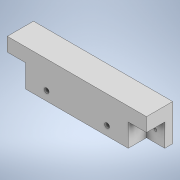
# Autodesk Inventor part: side_bumper_upper
Saved by Autodesk Inventor 2020 (Build 240168000, 168)
## iProperties
Created: 2022-07-20
Part Number: side_bumper_upper
Material: 일반
Document SubType Name: Modeling
Designer: SeungJin
Density: 1 g/cm^3
Appearance: 기본값
Author: SeungJin
Autodesk Inventor part; units mm, degrees
ref_plane "YZ Plane" through (0, 0, 0) normal (1, 0, 0) x (0, 1, 0)
ref_plane "XZ Plane" through (0, 0, 0) normal (0, 1, 0) x (-1, 0, 0)
ref_plane "XY Plane" through (0, 0, 0) normal (0, 0, 1) x (1, 0, 0)
ref_plane "작업 평면1" through (-180.5399, 22.5444, -43) normal (0, 0, 1) x (1, 0, 0)
sketch "스케치3" plane through (-180.5399, 22.5444, -43) normal (0, 0, 1) x (1, 0, 0)
  line L0 (146.4615, -22.6) -> (144.383, -19) projected
  line L1 (144.383, -19) -> (146.4615, -15.4) projected
  line L2 (146.4615, -15.4) -> (150.6184, -15.4) projected
  line L3 (150.6184, -15.4) -> (152.6968, -19) projected
  line L4 (152.6968, -19) -> (150.6184, -22.6) projected
  line L5 (150.6184, -22.6) -> (146.4615, -22.6) projected
  line L6 (45.113, -19) -> (47.1915, -15.4) projected
  line L7 (47.1915, -15.4) -> (51.3484, -15.4) projected
  line L8 (51.3484, -15.4) -> (53.4269, -19) projected
  line L9 (53.4269, -19) -> (51.3484, -22.6) projected
  line L10 (51.3484, -22.6) -> (47.1915, -22.6) projected
  line L11 (47.1915, -22.6) -> (45.113, -19) projected
  circle A0 centre (34.635, -45) radius 2.25 projected
  circle A1 centre (133.9049, -45) radius 2.25 projected
  line L12 (168.5399, -60) -> (0, -60) projected
  line L13 (198.5399, -22.5444) -> (168.5399, -22.5444) projected
  line L14 (168.5399, -22.5444) -> (168.5399, -60) projected
  line L15 (198.5399, 0) -> (198.5399, -22.5444) projected
  line L16 (0, 0) -> (198.5399, 0) projected
  line L17 (0, -60) -> (0, 0) projected
  line L18 (0, 0) -> (-30, 0)
  line L19 (-30, 0) -> (-30, -60)
  line L20 (-30, -60) -> (0, -60)
  line L21 (0, -60) -> (0, 0)
  line L22 (69.27, -22.5444) -> (69.27, -60)
  line L23 (69.27, -60) -> (99.27, -60)
  line L24 (168.5399, -22.5444) -> (168.5399, -60) projected
  line L25 (168.5399, -60) -> (198.5399, -60)
  line L26 (198.5399, -60) -> (198.5399, -22.5444)
  point P0 (180.5399, -22.5444)
  dimension "d10" = 30
  constraints: 16 end point, 2 parallel, 2 perpendicular, 1 horizontal, 1 point on line
  measures "d10" distance of L20.end L19.end
extrude "돌출3" add sketch "스케치3" along normal blind 13 contours L0 L1 L2 L3 L4 L5 | L6 L7 L8 L9 L10 L11 | A0 | A1 | L12 L17 L16 L15 L13 L14 | L14 L13 L26 L25 | L20 L19 L18 L17
ref_plane "작업 평면2" through (-180.5399, 22.5444, -30) normal (0, 0, 1) x (1, 0, 0)
sketch "스케치4" plane through (-180.5399, 22.5444, -30) normal (0, 0, 1) x (1, 0, 0)
  line L0 (198.5399, 0) -> (-30, 0) projected
  line L1 (-30, 0) -> (-30, -60) projected
  line L2 (-30, -60) -> (198.5399, -60) projected
  line L3 (198.5399, -60) -> (198.5399, 0) projected
  line L4 (198.5399, 0) -> (-30, 0) projected
  line L5 (-30, 0) -> (0, 0)
  line L6 (0, 0) -> (0, -22.544)
  line L7 (0, -22.544) -> (-30, -22.544)
  line L8 (-30, -22.544) -> (-30, 0)
  line L9 (0, 0) -> (198.5399, 0) projected
  line L10 (198.5399, 0) -> (168.5399, 0)
  line L11 (168.5399, 0) -> (168.5399, -22.544)
  line L12 (168.5399, -22.544) -> (198.5399, -22.544)
  line L13 (198.5399, -22.544) -> (198.5399, 0)
  line L14 (0, -60) -> (0, -10) projected
  line L15 (0, -22.544) -> (0, -60)
  line L16 (168.5399, -22.5444) -> (168.5399, -60) projected
  line L17 (168.5399, -22.544) -> (168.5399, -60)
  point P0 (180.5399, -22.5444)
  dimension "d13" = 30
  dimension "d14" = 22.544
  dimension "d15" = 22.544
  constraints: 20 end point, 2 horizontal, 2 parallel, 1 collinear, 1 perpendicular, 1 vertical
  measures "d13" distance of L6.end L7.end
  measures "d14" distance of L5.end L6.end
  measures "d15" distance of L11.end L10.end
extrude "돌출4" add sketch "스케치4" along normal blind 30 contours L3 L12 L11 L0 | L11 L16 L2 L14 L6 L0 | L6 L7 L1 L0
sketch "스케치5" plane through (-180.5399, 22.5444, 0) normal (0, 0, 1) x (1, 0, 0)
  line L0 (-30, -22.544) -> (0, -22.544) projected
  line L1 (0, -22.544) -> (0, -60) projected
  line L2 (0, -60) -> (168.5399, -60) projected
  line L3 (168.5399, -60) -> (168.5399, -22.544) projected
  line L4 (168.5399, -22.544) -> (198.5399, -22.544) projected
  line L5 (198.5399, -22.544) -> (198.5399, 0) projected
  line L6 (198.5399, 0) -> (-30, 0) projected
  line L7 (-30, 0) -> (-30, -22.544) projected
  circle A0 centre (34.635, -45) radius 2.25 projected
  line L8 (30.4781, -45) -> (32.5565, -48.6) projected
  line L9 (32.5565, -41.4) -> (30.4781, -45) projected
  line L10 (36.7134, -41.4) -> (32.5565, -41.4) projected
  line L11 (38.7919, -45) -> (36.7134, -41.4) projected
  line L12 (36.7134, -48.6) -> (38.7919, -45) projected
  line L13 (32.5565, -48.6) -> (36.7134, -48.6) projected
  circle A1 centre (133.9049, -45) radius 2.25 projected
  line L14 (131.8265, -48.6) -> (135.9834, -48.6) projected
  line L15 (129.748, -45) -> (131.8265, -48.6) projected
  line L16 (131.8265, -41.4) -> (129.748, -45) projected
  line L17 (135.9834, -41.4) -> (131.8265, -41.4) projected
  line L18 (138.0619, -45) -> (135.9834, -41.4) projected
  line L19 (135.9834, -48.6) -> (138.0619, -45) projected
  circle A2 centre (133.9049, -45) radius 2.25 projected
  point P0 (180.5399, -22.5444)
  constraints: 2 coincident
hole "구멍1" at (-46.635, -22.4556, 0) at (-145.9049, -22.4556, 0) direction (0, 0, -1) diameter 4.5 end through all counterbore diameter 8 counterbore depth 25 clearance for "Hex Head Cap Screw ISO 24017" size "M4" standard "ISO"
ref_plane "작업 평면4" through (-180.5399, 22.5444, -43) normal (0, 0, -1) x (-1, 0, 0)
sketch "스케치6" plane through (-180.5399, 22.5444, -43) normal (0, 0, -1) x (-1, 0, 0)
  line L0 (-198.5399, -60) -> (-198.5399, 0) projected
  line L1 (30, -60) -> (-198.5399, -60) projected
  line L2 (30, -60) -> (-198.5399, -60) projected
  line L3 (30, 0) -> (30, -60) projected
  line L4 (-198.5399, 0) -> (30, 0) projected
  line L5 (-198.5399, -60) -> (-198.5399, 0) projected
  line L6 (30, 0) -> (30, -60) projected
  line L7 (-198.5399, 0) -> (30, 0) projected
  point P0 (-180.5399, -22.5444)
  point P1 (-183.5399, -41.2722)
  point P2 (15, -41.2722)
hole "구멍2" at (3, -18.7278, -43) at (-195.5399, -18.7278, -43) direction (0, 0, 1) diameter 4.5 end through all counterbore diameter 8 counterbore depth 5 clearance for "Hex Head Cap Screw ISO 24017" size "M4" standard "ISO"
